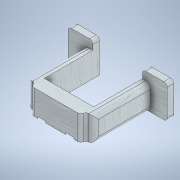
# Autodesk Inventor part: podstawa 01-3
Saved by Autodesk Inventor 2021 (Build 250183000, 183)
## iProperties
Created: 2021-11-05
Part Number: podstawa 01-3
Material: Generic
Document SubType Name: Modeling
Designer: Łukasz
Density: 1 g/cm^3
Appearance: Wood - Painted White
Author: Łukasz
Autodesk Inventor part; units mm, degrees
ref_plane "YZ Plane" through (0, 0, 0) normal (1, 0, 0) x (0, 1, 0)
ref_plane "XZ Plane" through (0, 0, 0) normal (0, 1, 0) x (-1, 0, 0)
ref_plane "XY Plane" through (0, 0, 0) normal (0, 0, 1) x (1, 0, 0)
sketch "Sketch1" plane through (0, 0, 0) normal (0, 0, 1) x (1, 0, 0)
  line L0 (0, 0) -> (40, 0)
  line L1 (40, 0) -> (40, -15)
  line L2 (40, -15) -> (0, -15)
  line L3 (0, -15) -> (0, 0)
  dimension "d0" = 40
  dimension "d1" = 15
  constraints: 8 end point, 2 parallel, 1 horizontal, 1 perpendicular
  measures "d0" distance of L1.end L2.end
  measures "d1" distance of L0.end L1.end
extrude "Extrusion1" add sketch "Sketch1" along normal blind 5
sketch "Sketch2" plane through (0, 0, 5) normal (0, 0, 1) x (1, 0, 0)
  line L0 (40, 0) -> (0, 0) projected
  line L1 (5, 0) -> (35, 0)
  line L2 (35, 0) -> (35, -15)
  line L3 (35, -15) -> (5, -15)
  line L4 (5, -15) -> (5, 0)
  line L5 (0, 0) -> (0, -15) projected
  dimension "d4" = 30
  dimension "d5" = 15
  dimension "d6" = 5
  constraints: 8 end point, 2 parallel, 1 horizontal, 1 perpendicular, 1 point on line
  measures "d4" distance of L2.end L3.end
  measures "d5" distance of L1.end L2.end
  measures "d6" distance between parallel lines of L5 L4
extrude "Extrusion2" add sketch "Sketch2" along normal blind 3
fillet "Fillet1" radius 2 4 edges at (35, -7.5, 5) (35, -7.5, 8) (5, -7.5, 5) (5, -7.5, 8)
sketch "Sketch3" plane through (0, 0, 0) normal (0, 0, -1) x (-1, 0, 0)
  line L0 (0, 0) -> (0, -15) projected
  line L1 (-40, 0) -> (0, 0) projected
  line L2 (0, -15) -> (-5, -15)
  line L3 (-5, -15) -> (-5, 0)
  line L4 (-5, 0) -> (0, 0)
  line L5 (0, 0) -> (0, -15)
  line L6 (-40, -15) -> (-40, 0) projected
  line L7 (0, -15) -> (-40, -15) projected
  line L8 (-40, 0) -> (-35, 0)
  line L9 (-35, 0) -> (-35, -15)
  line L10 (-35, -15) -> (-40, -15)
  line L11 (-40, -15) -> (-40, 0)
  dimension "d10" = 5
  dimension "d11" = 5
  constraints: 16 end point, 4 parallel, 2 horizontal, 2 perpendicular, 2 point on line
  measures "d10" distance of L3.end L4.end
  measures "d11" distance of L9.end L10.end
extrude "Extrusion3" add sketch "Sketch3" along normal blind 33.5 contours L0 L2 L3 L1 | L9 L7 L6 L1
sketch "Sketch4" plane through (0, 0, -33.5) normal (0, 0, -1) x (-1, 0, 0)
  line L0 (-35, 0) -> (-35, -15) projected
  line L1 (-35, -15) -> (-50, -15)
  line L2 (-50, -15) -> (-50, 5)
  line L3 (-50, 5) -> (-35, 5)
  line L4 (-35, 5) -> (-35, -15)
  line L5 (-5, -15) -> (-35, -15) projected
  line L6 (-5, -15) -> (10, -15)
  line L7 (10, -15) -> (10, 5)
  line L8 (10, 5) -> (-5, 5)
  line L9 (-5, 5) -> (-5, -15)
  point P0 (-4.9365, 0)
  dimension "d18" = 15
  dimension "d19" = 20
  dimension "d20" = 15
  constraints: 16 end point, 4 parallel, 2 horizontal, 2 perpendicular, 1 point on line
  measures "d18" distance of L2.end L3.end
  measures "d19" distance of L1.end L2.end
  measures "d20" distance of L8.end L7.end
extrude "Extrusion4" add sketch "Sketch4" against normal blind 4
fillet "Fillet2" radius 3 6 edges at (0, 0, -12.25) (0, -7.5, 5) (0, -15, -12.25) (40, -15, -12.25) (40, -7.5, 5) (40, 0, -12.25)
fillet "Fillet3" radius 2 6 edges at (-10, 5, -31.5) (5, 5, -31.5) (-10, -15, -31.5) (35, 5, -31.5) (50, 5, -31.5) (50, -15, -31.5)
sketch "Sketch5" plane through (6.873, -15, 8) normal (0, -1, 0) x (1, 0, 0)
  arc A0 (2.2162, 0) -> (7.038, 0) centre (4.6271, -3.5) ccw
  arc A1 (19.2162, 0) -> (24.038, 0) centre (21.6271, -3.5) ccw
  line L0 (-1.8729, -41.5) -> (-14.8729, -41.5)
  line L1 (-14.8729, -37.5) -> (-3.8729, -37.5)
  line L2 (-16.8729, -37.5) -> (-16.8729, -41.5)
  line L3 (-6.8729, -6) -> (-6.8729, -37.5)
  arc A2 (0.0001, 0) -> (-1.9364, -1.5) centre (0.0001, -2) ccw
  arc A3 (-3.8729, -3) -> (-1.9364, -1.5) centre (-3.8729, -1) ccw
  arc A4 (-3.8729, -3) -> (-6.8729, -6) centre (-3.8729, -6) ccw
  line L4 (0, 0) -> (26.254, 0) projected
  point P0 (-6.873, -8)
  point P1 (-1.8729, -43)
  constraints: 10 point on circle, 8 end point, 5 centre point
extrude "Extrusion5" cut sketch "Sketch5" against normal blind 1
sketch "Sketch6" plane through (5, -15, 0) normal (0, -1, 0) x (1, 0, 0)
  arc A0 (21.0892, 8) -> (25.911, 8) centre (23.5001, 4.5) ccw projected
  circle A1 centre (23.5001, 4.5) radius 0.75
  arc A2 (4.0892, 8) -> (8.911, 8) centre (6.5001, 4.5) ccw projected
  circle A3 centre (6.5001, 4.5) radius 0.75
  point P0 (-5, 0)
  dimension "d27" = 1.5
  dimension "d28" = 1.5
  constraints: 2 centre point, 2 coincident
  measures "d27" diameter of A1
  measures "d28" diameter of A3
extrude "Extrusion6" cut sketch "Sketch6" against normal blind 10
body "Solid1"
